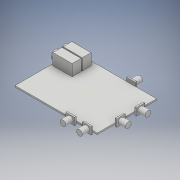
# Autodesk Inventor part: ADF41020-EVB
Saved by Autodesk Inventor 2018 (Build 220112000, 112)
## iProperties
Created: 2018-01-02
Part Number: ADF41020-EVB
Material: Generic
Document SubType Name: Modeling
Designer: rwradema
Density: 1 g/cm^3
Appearance: Default
Author: rwradema
Autodesk Inventor part; units mm, degrees
ref_plane "YZ Plane" through (0, 0, 0) normal (1, 0, 0) x (0, 1, 0)
ref_plane "XZ Plane" through (0, 0, 0) normal (0, 1, 0) x (-1, 0, 0)
ref_plane "XY Plane" through (0, 0, 0) normal (0, 0, 1) x (1, 0, 0)
sketch "Sketch1" plane through (0, 0, 0) normal (0, 0, 1) x (1, 0, 0)
  line L0 (-45, 32.5) -> (45, 32.5)
  line L1 (45, 32.5) -> (45, -32.5)
  line L2 (45, -32.5) -> (-45, -32.5)
  line L3 (-45, -32.5) -> (-45, 32.5)
  line L4 (-45, 32.5) -> (45, -32.5) construction
  line L5 (45, 32.5) -> (-45, -32.5) construction
  point P0 (0, 0)
  dimension "d0" = 90
  dimension "d1" = 65
  constraints: 12 end point, 2 midpoint, 2 parallel, 1 horizontal, 1 perpendicular
  measures "d0" distance of L0.start L0.end
  measures "d1" distance of L2.end L0.start
extrude "Extrusion1" add sketch "Sketch1" along normal blind 1.6
sketch "Sketch2" plane through (0, 0, 1.6) normal (0, 0, 1) x (1, 0, 0)
  point P0 (0, 0)
sketch "Sketch3" plane through (-45, 32.5, 0) normal (0, 1, 0) x (1, 0, 0)
  point P0 (45, 0)
sketch "Sketch4" plane through (-45, 32.5, 0) normal (0, 1, 0) x (1, 0, 0)
  line L0 (57.225, -5.6) -> (66.775, -5.6)
  line L1 (66.775, -5.6) -> (66.775, 2.4)
  line L2 (66.775, 2.4) -> (57.225, 2.4)
  line L3 (57.225, 2.4) -> (57.225, -5.6)
  line L4 (90, -1.6) -> (0, -1.6) projected
  line L5 (57.225, -5.6) -> (66.775, 2.4) construction
  line L6 (66.775, -5.6) -> (57.225, 2.4) construction
  point P0 (45, 0)
  point P1 (62, -1.6)
  dimension "d4" = 9.55
  dimension "d5" = 8
  dimension "d8" = 62
  constraints: 12 end point, 2 midpoint, 2 parallel, 1 horizontal, 1 perpendicular, 1 point on line
  measures "d4" distance of L0.start L0.end
  measures "d5" distance of L2.end L0.start
  measures "d8" distance of L4.end point (62, -1.6)
extrude "Extrusion2" add sketch "Sketch4" along normal blind 1.55
sketch "Sketch5" plane through (45, -32.5, 0) normal (1, 0, 0) x (0, 0, -1)
  line L0 (-5.6, 50.775) -> (2.4, 50.775)
  line L1 (2.4, 50.775) -> (2.4, 41.225)
  line L2 (2.4, 41.225) -> (-5.6, 41.225)
  line L3 (-5.6, 41.225) -> (-5.6, 50.775)
  line L4 (-1.6, 0) -> (-1.6, 65) projected
  line L5 (-5.6, 50.775) -> (2.4, 41.225) construction
  line L6 (2.4, 50.775) -> (-5.6, 41.225) construction
  line L7 (-5.8505, 29.275) -> (2.1495, 29.275)
  line L8 (2.1495, 29.275) -> (2.1495, 19.725)
  line L9 (2.1495, 19.725) -> (-5.8505, 19.725)
  line L10 (-5.8505, 19.725) -> (-5.8505, 29.275)
  line L11 (-5.8505, 29.275) -> (2.1495, 19.725) construction
  line L12 (2.1495, 29.275) -> (-5.8505, 19.725) construction
  point P0 (0, 32.5)
  point P1 (-1.6, 46)
  point P2 (-1.8505, 24.5)
  dimension "d9" = 9.55
  dimension "d10" = 8
  dimension "d11" = 19
  dimension "d12" = 24.5
  constraints: 24 end point, 6 parallel, 4 midpoint, 2 horizontal, 2 perpendicular, 1 point on line
  measures "d9" distance of L2.end L0.start
  measures "d10" distance of L0.start L0.end
  measures "d11" distance of point (-1.6, 46) L4.end
  measures "d12" vertical distance of L4.start point (-1.851, 24.5)
extrude "Extrusion3" add sketch "Sketch5" along normal blind 1.55
sketch "Sketch6" plane through (-45, -32.5, 0) normal (0, -1, 0) x (1, 0, 0)
  line L0 (66.775, 5.6091) -> (57.225, 5.6091)
  line L1 (57.225, 5.6091) -> (57.225, -2.3909)
  line L2 (57.225, -2.3909) -> (66.775, -2.3909)
  line L3 (66.775, -2.3909) -> (66.775, 5.6091)
  line L4 (66.775, 5.6091) -> (57.225, -2.3909) construction
  line L5 (57.225, 5.6091) -> (66.775, -2.3909) construction
  line L6 (84.775, 5.6) -> (75.225, 5.6)
  line L7 (75.225, 5.6) -> (75.225, -2.4)
  line L8 (75.225, -2.4) -> (84.775, -2.4)
  line L9 (84.775, -2.4) -> (84.775, 5.6)
  line L10 (0, 1.6) -> (90, 1.6) projected
  line L11 (84.775, 5.6) -> (75.225, -2.4) construction
  line L12 (75.225, 5.6) -> (84.775, -2.4) construction
  point P0 (45, 0)
  point P1 (62, 1.6091)
  point P2 (80, 1.6)
  dimension "d15" = 10
  dimension "d16" = 28
  dimension "d17" = 8
  dimension "d18" = 9.55
  constraints: 24 end point, 6 parallel, 4 midpoint, 2 horizontal, 2 perpendicular, 1 point on line
  measures "d15" distance of point (80, 1.6) L10.end
  measures "d16" distance of L10.end point (62, 1.609)
  measures "d17" distance of L8.end L6.start
  measures "d18" distance of L7.end L8.end
extrude "Extrusion4" add sketch "Sketch6" along normal blind 1.55
sketch "Sketch7" plane through (0, 0, 1.6) normal (0, 0, 1) x (1, 0, 0)
  line L0 (-43, 27.7) -> (-22, 27.7)
  line L1 (-22, 27.7) -> (-22, 17.95)
  line L2 (-22, 17.95) -> (-43, 17.95)
  line L3 (-43, 17.95) -> (-43, 27.7)
  line L4 (-43, 27.7) -> (-22, 17.95) construction
  line L5 (-22, 27.7) -> (-43, 17.95) construction
  line L6 (-43, 16.75) -> (-22, 16.75)
  line L7 (-22, 16.75) -> (-22, 7)
  line L8 (-22, 7) -> (-43, 7)
  line L9 (-43, 7) -> (-43, 16.75)
  line L10 (-43, 16.75) -> (-22, 7) construction
  line L11 (-22, 16.75) -> (-43, 7) construction
  line L12 (12.225, 32.5) -> (-45, 32.5) projected
  line L13 (-45, 32.5) -> (-45, -32.5) projected
  point P0 (0, 0)
  point P1 (-32.5, 22.825)
  point P2 (-32.5, 11.875)
  dimension "d21" = 21
  dimension "d22" = 9.75
  dimension "d23" = 25.5
  dimension "d24" = 4.8
  dimension "d25" = 2
  constraints: 24 end point, 4 midpoint, 4 parallel, 2 equal length, 2 horizontal, 2 perpendicular, 1 point on line
  measures "d21" distance of L0.start L0.end
  measures "d22" distance of L0.end L1.end
  measures "d23" distance between parallel lines of L12 L8
  measures "d24" distance between parallel lines of L12 L0
  measures "d25" distance between parallel lines of L13 L9
extrude "Extrusion5" add sketch "Sketch7" along normal blind 12.6
sketch "Sketch8" plane through (-43, 17.95, 1.6) normal (-1, 0, 0) x (0, 0, 1)
  circle A0 centre (7.3783, 4.875) radius 4.5
  circle A1 centre (7.3783, -6.0762) radius 4.5
  point P0 (-1.6, -17.95)
  dimension "d28" = 9
  constraints: 2 centre point, 1 equal radius
  measures "d28" diameter of A0
extrude "Extrusion6" add sketch "Sketch8" along normal blind 2.4
sketch "Sketch9" plane through (-45, -34.05, 0) normal (0, -1, 0) x (1, 0, 0)
  line L0 (66.775, 5.6091) -> (57.225, 5.6091) construction
  line L1 (62, 5.6091) -> (62, -2.3909) construction
  line L2 (57.225, -2.3909) -> (66.775, -2.3909) construction
  line L3 (57.225, 1.6) -> (66.775, 1.6) construction
  line L4 (57.225, 1.6) -> (66.775, 1.6) construction
  line L5 (84.775, 5.6) -> (75.225, 5.6) construction
  line L6 (80, 5.6) -> (80, -3.4898) construction
  line L7 (75.225, 0) -> (75.225, 1.6) construction
  line L8 (75.225, 1.6) -> (84.775, 1.6) construction
  line L9 (75.225, 1.6) -> (84.775, 1.6) construction
  circle A0 centre (62, 1.6) radius 3.125
  circle A1 centre (80, 1.6) radius 3.125
  point P0 (45, 0)
  dimension "d31" = 6.25
  constraints: 8 end point, 5 midpoint, 2 centre point, 2 collinear, 1 equal radius, 1 vertical
  measures "d31" diameter of A1
extrude "Extrusion7" add sketch "Sketch9" along normal blind 8
sketch "Sketch10" plane through (46.55, -32.5, 0) normal (1, 0, 0) x (0, 0, -1)
  line L0 (-5.6, 50.775) -> (-5.6, 41.225) construction
  line L1 (-5.6, 46) -> (2.4, 46) construction
  line L2 (2.4, 41.225) -> (2.4, 50.775) construction
  line L3 (-5.8505, 29.275) -> (-5.8505, 19.725) construction
  line L4 (-5.8505, 24.5) -> (2.1495, 24.5) construction
  line L5 (2.1495, 29.275) -> (2.1495, 19.725) construction
  line L6 (-1.6, 50.775) -> (0, 50.775) construction
  line L7 (-1.6, 39.5) -> (-1.6, 49.25) construction
  line L8 (-1.6, 50.775) -> (-1.6, 39.5) construction
  line L9 (-1.6, 65) -> (-1.6, 0) construction
  line L10 (-1.6, 29.275) -> (-1.6, 19.725) construction
  circle A0 centre (-1.6, 46) radius 3.125
  circle A1 centre (-1.6, 24.5) radius 3.125
  point P0 (0, 32.5)
  dimension "d34" = 6.25
  constraints: 8 end point, 6 midpoint, 2 centre point, 1 collinear, 1 equal radius, 1 point on line, 5 other
  measures "d34" diameter of A0
extrude "Extrusion8" add sketch "Sketch10" along normal blind 8
sketch "Sketch11" plane through (-45, 34.05, 0) normal (0, 1, 0) x (1, 0, 0)
  line L0 (66.775, -5.6091) -> (57.225, -5.6091) construction
  line L1 (62, -5.6091) -> (62, 2.3909) construction
  line L2 (57.225, 2.3909) -> (66.775, 2.3909) construction
  line L3 (57.225, -1.6) -> (66.775, -1.6) construction
  line L4 (57.225, -1.6) -> (66.775, -1.6) construction
  circle A0 centre (62, -1.6) radius 3.125
  point P0 (45, 0)
  dimension "d37" = 6.25
  constraints: 4 end point, 3 midpoint, 1 centre point, 1 collinear
  measures "d37" diameter of A0
extrude "Extrusion9" add sketch "Sketch11" along normal blind 8
body "Solid1"
